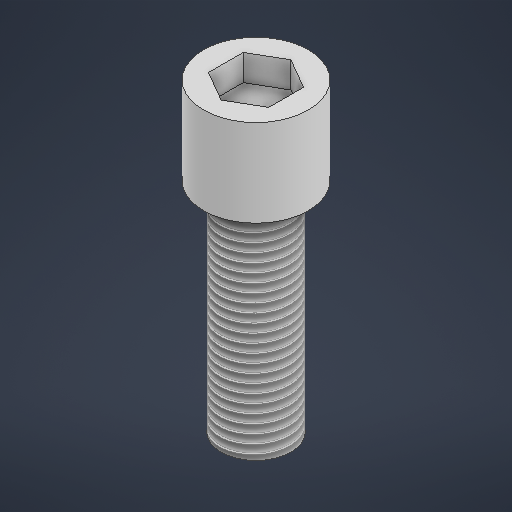
# Autodesk Inventor part: 4mm_0.5_Screw
Saved by Autodesk Inventor 2026.2 (Build 302298000, 298)
## iProperties
Created: 2025-12-16
Part Number: 4mm_0.5_Screw
Material: Generic
Document SubType Name: Modeling
Designer: Thoma
Density: 1 g/cm^3
Appearance: Default
Author: Thoma
Autodesk Inventor part; units mm, degrees
ref_plane "YZ Plane" through (0, 0, 0) normal (1, 0, 0) x (0, 1, 0)
ref_plane "XZ Plane" through (0, 0, 0) normal (0, 1, 0) x (-1, 0, 0)
ref_plane "XY Plane" through (0, 0, 0) normal (0, 0, 1) x (1, 0, 0)
sketch "Sketch1" plane through (0, 0, 0) normal (0, 1, 0) x (-1, 0, 0)
  circle A0 centre (0, 0) radius 2
  dimension "d0" = 4
  constraints: 1 centre point, 1 coincident
  measures "d0" diameter of A0
extrude "Extrusion1" add sketch "Sketch1" along normal blind 12.5
sketch "Sketch2" plane through (0, 12.5, 0) normal (0, 1, 0) x (1, 0, 0)
  circle A0 centre (0, 0) radius 3
  dimension "d3" = 6
  constraints: 1 centre point, 1 coincident
  measures "d3" diameter of A0
extrude "Extrusion2" add sketch "Sketch2" along normal blind 5
sketch "Sketch3" plane through (0, 17.5, 0) normal (0, 1, 0) x (1, 0, 0)
  circle A0 centre (0, 0) radius 2 projected
  line L0 (0, 2) -> (1.7321, 1)
  line L1 (1.7321, 1) -> (1.7321, -1)
  line L2 (1.7321, -1) -> (0, -2)
  line L3 (0, -2) -> (-1.7321, -1)
  line L4 (-1.7321, -1) -> (-1.7321, 1)
  line L5 (-1.7321, 1) -> (0, 2)
  constraints: 12 end point, 1 coincident, 1 vertical alignment, 14 other
extrude "Extrusion3" cut sketch "Sketch3" against normal blind 1.5 contours L1 L2 L3 L4 L5 L0
thread "Thread1" size "M4x0.5" class "6g" standard "ANSI Metric M Profile" length 20
body "Solid1"
